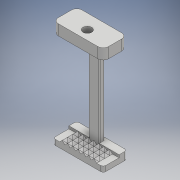
# Autodesk Inventor part: Clamp-part1-Base9x19mm-narrowTOP-maxSample28mm
Saved by Autodesk Inventor 2017 (Build 210142000, 142)
## iProperties
Created: 2021-08-04
Part Number: Clamp-part1-Base9x19mm-narrowTOP-maxSample28mm
Material: Generic
Document SubType Name: Modeling
Designer: Nikita
Density: 1 g/cm^3
Appearance: Default
Author: Nikita
Autodesk Inventor part; units mm, degrees
ref_plane "YZ Plane" through (0, 0, 0) normal (1, 0, 0) x (0, 1, 0)
ref_plane "XZ Plane" through (0, 0, 0) normal (0, 1, 0) x (-1, 0, 0)
ref_plane "XY Plane" through (0, 0, 0) normal (0, 0, 1) x (1, 0, 0)
sketch "Sketch1" plane through (0, 0, 0) normal (0, 0, 1) x (1, 0, 0)
  line L0 (0, 0) -> (19, 0)
  line L1 (19, 0) -> (19, 9)
  line L2 (19, 9) -> (0, 9)
  line L3 (0, 9) -> (0, 0)
  point P0 (9.5, 9)
  dimension "d0" = 19
  dimension "d1" = 9
  constraints: 8 end point, 2 parallel, 1 horizontal, 1 midpoint, 1 perpendicular
  measures "d0" distance of L2.end L1.end
  measures "d1" distance of L1.end L0.end
extrude "Extrusion1" add sketch "Sketch1" along normal blind 3
sketch "Sketch2" plane through (0, 0, 3) normal (0, 0, 1) x (1, 0, 0)
  line L0 (19, 9) -> (0, 9) projected
  circle A0 centre (9.5, 7) radius 1
  point P0 (0, 0)
  point P1 (9.5, 9)
  dimension "d4" = 2
  dimension "d5" = 2
  constraints: 1 centre point, 1 midpoint
  measures "d4" diameter of A0
  measures "d5" distance from line of A0.centre L0
extrude "Extrusion2" add sketch "Sketch2" along normal blind 1.5
sketch "Sketch6" plane through (9.5, 7, 4.5) normal (0, 0, 1) x (1, 0, 0)
  circle A0 centre (0, 0) radius 1 projected
  line L0 (2, -1) -> (-2, -1)
  line L1 (-2, -1) -> (-2, 1)
  line L2 (-2, 1) -> (2, 1)
  line L3 (2, 1) -> (2, -1)
  line L4 (2, -1) -> (-2, 1) construction
  line L5 (-2, -1) -> (2, 1) construction
  point P0 (-9.5, -7)
  dimension "d13" = 4
  constraints: 12 end point, 2 midpoint, 2 parallel, 1 coincident, 1 horizontal, 1 perpendicular
  measures "d13" distance of L1.end L2.end
extrude "Extrusion5" add sketch "Sketch6" along normal blind 32
sketch "Sketch7" plane through (9.5, 7, 36.5) normal (0, 0, 1) x (1, 0, 0)
  circle A0 centre (0, 0) radius 1 projected
  line L0 (-9.5, -7) -> (9.5, -7) projected
  line L1 (9.5, -7) -> (9.5, 2) projected
  line L2 (9.5, 2) -> (-9.5, 2) projected
  line L3 (-9.5, 2) -> (-9.5, -7) projected
  arc A1 (0, -1) -> (0, 1) centre (0, 0) ccw projected
  arc A2 (0, 1) -> (0, -1) centre (0, 0) ccw projected
extrude "Extrusion6" add sketch "Sketch7" along normal blind 4 contours A0 | L3 L2 L1 L0
sketch "Sketch8" plane through (9.5, 7, 40.5) normal (0, 0, 1) x (1, 0, 0)
  line L0 (-9.5, -7) -> (9.5, -7) projected
  line L1 (9.5, -7) -> (9.5, 2) projected
  line L2 (9.5, 2) -> (-9.5, 2) projected
  line L3 (-9.5, 2) -> (-9.5, -7) projected
  circle A0 centre (0, -3.5) radius 1.65
  dimension "d18" = 3.3
  dimension "d66" = 5.5
  constraints: 1 centre point
  measures "d18" diameter of A0
  measures "d66" distance from line of A0.centre L2
extrude "Extrusion7" cut sketch "Sketch8" against normal blind 4 contours A0
sketch "Sketch10" plane through (0, 0, 0) normal (-1, 0, 0) x (0, 0, 1)
  line L0 (0, 0) -> (3, 0) projected
  line L1 (3, 9) -> (3, 0) projected
  line L2 (3, 0) -> (2, 0)
  line L3 (2, 0) -> (2, 6)
  line L4 (2, 6) -> (3, 6)
  line L5 (3, 6) -> (3, 0)
  line L6 (3, 0) -> (2, 1)
  line L7 (3, 0) -> (4.4142, 0) construction
  line L8 (2, 1) -> (3, 2)
  line L9 (3, 0) -> (3, 9) projected
  line L10 (3, 2) -> (2, 3)
  line L11 (2, 3) -> (3, 4)
  line L12 (2, 5) -> (3, 4)
  line L13 (2, 5) -> (3, 6)
  dimension "d23" = 1
  dimension "d24" = 6
  dimension "d25" = 135
  dimension "d26" = 90
  constraints: 22 end point, 4 point on line, 3 perpendicular, 2 horizontal, 2 parallel, 1 equal length, 1 midpoint
  measures "d23" distance of L3.end L4.end
  measures "d24" distance of L2.end L3.end
  measures "d25" angle of L7 L6
  measures "d26" angle of L6 L8
extrude "Extrusion8" cut sketch "Sketch10" against normal up to next contours L6 L8 L1 | L10 L11 L1 | L12 L13 L1
sketch "Sketch11" plane through (0, 0, 0) normal (0, -1, 0) x (1, 0, 0)
  line L0 (0, 3) -> (9.5, 3) projected
  line L1 (0, 3) -> (19, 3)
  line L2 (19, 3) -> (19, 2)
  line L3 (19, 2) -> (8.5, 2)
  line L4 (0, 2) -> (0, 3)
  line L5 (0, 3) -> (0, 2) projected
  line L6 (0, 3) -> (1.4142, 3) construction
  line L7 (19, 3) -> (0, 3) projected
  line L8 (9.5, 3) -> (8.5, 2)
  line L9 (9.5, 3) -> (10.9142, 3) construction
  line L10 (10.5, 2) -> (8.5, 2)
  line L11 (9.5, 3) -> (10.5, 2)
  line L12 (10.5, 2) -> (8.5, 2)
  line L13 (8.5, 2) -> (0, 2)
  line L14 (7.5, 3) -> (8.5, 2)
  line L15 (8.5, 2) -> (6.5, 2)
  line L16 (7.5, 3) -> (6.5, 2)
  line L17 (5.5, 3) -> (6.5, 2)
  line L18 (6.5, 2) -> (4.5, 2)
  line L19 (5.5, 3) -> (4.5, 2)
  line L20 (3.5, 3) -> (4.5, 2)
  line L21 (4.5, 2) -> (2.5, 2)
  line L22 (3.5, 3) -> (2.5, 2)
  line L23 (12.5, 2) -> (10.5, 2)
  line L24 (11.5, 3) -> (12.5, 2)
  line L25 (11.5, 3) -> (10.5, 2)
  line L26 (14.5, 2) -> (12.5, 2)
  line L27 (13.5, 3) -> (14.5, 2)
  line L28 (13.5, 3) -> (12.5, 2)
  line L29 (16.5, 2) -> (14.5, 2)
  line L30 (15.5, 3) -> (16.5, 2)
  line L31 (15.5, 3) -> (14.5, 2)
  point P0 (0, 0)
  dimension "d30" = 135
  dimension "d33" = 2
  dimension "d40" = 2
  constraints: 58 end point, 5 horizontal, 5 point on line, 3 collinear, 3 parallel, 2 perpendicular, 1 coincident, 1 equal length, 39 other
  measures "d30" angle of L8 L9
  measures "d33" distance of L8.start L14.start
  measures "d40" distance of L11.end L23.start
extrude "Extrusion9" cut sketch "Sketch11" against normal blind 6 contours L0 L22 L13 L4 | L0 L19 L20 | L0 L16 L17 | L0 L8 L14 | L1 L25 L11 | L1 L28 L24 | L1 L31 L27 | L1 L2 L3 L30
fillet "Fillet2" radius 1 4 edges at (19, 0, 1) (19, 9, 1.5) (0, 0, 1) (0, 9, 1.5)
fillet "Fillet3" radius 2 4 edges at (19, 0, 38.5) (19, 9, 38.5) (0, 0, 38.5) (0, 9, 38.5)
extrude "Extrusion10" add sketch "Sketch6" against normal up to surface (1.5 mm away) contours A0 L2 L3 L0 | A0 L0 L1 L2
sketch "Sketch12" plane through (9.5, 7, 36.5) normal (0, 0, -1) x (-1, 0, 0)
  circle A0 centre (0, 0) radius 1 projected
  line L0 (-2, 1) -> (-2, -1) projected
  line L1 (-2, -1) -> (2, -1) projected
  line L2 (2, 1) -> (-2, 1) projected
  line L3 (2, -1) -> (2, 1) projected
  point P0 (9.5, -7)
extrude "Extrusion11" cut sketch "Sketch12" along normal blind 4 contours A0 L2 L3 L1 | A0 L1 L0 L2
chamfer "Chamfer3" distance 2 distance2 1 1 edges at (7.5, 7, 32.5) measured on face at (7.5, 7, 32)
chamfer "Chamfer4" distance 2 distance2 1 1 edges at (11.5, 7, 32.5) measured on face at (11.5, 7, 32)
fillet "Fillet4" radius 0.3 4 edges at (11.5, 6, 16.7501) (7.5, 6, 16.7501) (11.5, 8, 16.7501) (7.5, 8, 16.7501)
body "Solid1"
